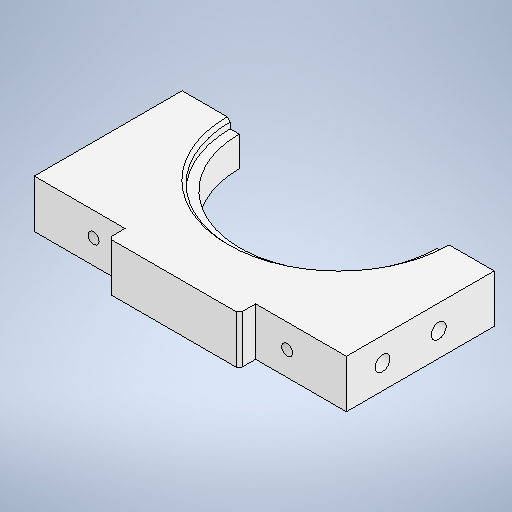
# Autodesk Inventor part: joint4_frame_2
Saved by Autodesk Inventor 2025.3 (Build 293356030, 356C)
## iProperties
Created: 2025-11-09
Part Number: joint4_frame_2
Material: PLA filament
Document SubType Name: Modeling
Designer: MSI
Mass: 66.0962 g
Surface Area: 141.432 cm^2
Volume: 55.0801 cm^3
Density: 1.2 g/cm^3
Appearance: 일반
Author: MSI
Autodesk Inventor part; units mm, degrees
ref_plane "YZ Plane" through (0, 0, 0) normal (1, 0, 0) x (0, 1, 0)
ref_plane "XZ Plane" through (0, 0, 0) normal (0, 1, 0) x (-1, 0, 0)
ref_plane "XY Plane" through (0, 0, 0) normal (0, 0, 1) x (1, 0, 0)
sketch "스케치1" plane through (0, 0, 0) normal (0, 1, 0) x (-1, 0, 0)
  line L0 (-104.5, 55) -> (104.5, 55)
  line L1 (104.5, 55) -> (104.5, -55)
  line L2 (104.5, -55) -> (-104.5, -55)
  line L3 (-104.5, -55) -> (-104.5, 55)
  line L4 (-104.5, 55) -> (104.5, -55) construction
  line L5 (104.5, 55) -> (-104.5, -55) construction
  point P0 (0, 0)
  dimension "d0" = 209
  dimension "d1" = 110
  constraints: 12 end point, 2 midpoint, 2 parallel, 1 horizontal, 1 perpendicular
  measures "d0" distance of L1.end L2.end
  measures "d1" distance of L0.end L1.end
extrude "돌출1" add sketch "스케치1" along normal mid plane 16
sketch "스케치2" plane through (0, 8, 0) normal (0, 1, 0) x (1, 0, 0)
  line L0 (-104.5, 55) -> (-104.5, -55) projected
  line L1 (-104.5, -40) -> (-94, -40)
  line L2 (-94, -40) -> (-94, 40)
  line L3 (-94, 40) -> (-104.5, 40)
  line L4 (-104.5, 40) -> (-104.5, -40)
  line L5 (-104.5, -55) -> (104.5, -55) projected
  point P0 (0, 0)
  point P1 (-94, 0)
  dimension "d4" = 10.5
  dimension "d5" = 15
  constraints: 8 end point, 2 parallel, 1 horizontal, 1 horizontal alignment, 1 midpoint, 1 perpendicular, 1 point on line
  measures "d4" distance of L2.end L3.end
  measures "d5" distance between parallel lines of L5 L1
extrude "돌출2" cut sketch "스케치2" against normal through all
sketch "스케치9" plane through (0, 8, 0) normal (0, 1, 0) x (1, 0, 0)
  line L0 (0, -0.25) -> (-158.4246, -0.25)
  line L1 (-158.4246, -0.25) -> (-158.4246, -70.8007)
  line L2 (-158.4246, -70.8007) -> (0, -70.8007)
  line L3 (0, -70.8007) -> (0, -0.25)
  point P0 (0, 0)
  dimension "d55" = 0.25
  constraints: 8 end point, 2 parallel, 1 horizontal, 1 perpendicular, 1 point on line
  measures "d55" distance from line of point (0, 0) L0
sketch "스케치10" plane through (-35.9991, 8, 0.25) normal (0, 0, -1) x (-1, 0, 0)
  line L0 (6.5004, -8) -> (29.0004, -8)
  line L1 (58.0009, 0) -> (0, 0) projected
  point P0 (-35.9991, -8)
  point P1 (29.0004, 0)
  point P2 (29.0004, 0)
  dimension "d66" = 22.5
  constraints: 2 coincident, 2 end point, 2 midpoint, 1 horizontal, 1 point on line, 1 vertical alignment
  measures "d66" distance of L0.start L0.end
mirror "미러1" about plane through (0, 0, 0) normal (1, 0, 0) of "돌출2"
sketch "스케치3" plane through (-94, 8, -40) normal (-1, 0, 0) x (0, 0, 1)
  line L0 (13.4, -8) -> (66.6, -8)
  point P0 (40, -8)
  point P1 (40, -8)
  point P2 (26.7, -8)
  point P3 (53.3, -8)
  dimension "d8" = 13.3
  dimension "d9" = 13.3
  dimension "d10" = 53.2
  constraints: 3 coincident, 2 end point, 2 point on line, 1 horizontal, 1 midpoint
  measures "d8" distance of point (26.7, -8) point (13.4, -8)
  measures "d9" distance of point (53.3, -8) point (66.6, -8)
  measures "d10" distance of L0.start L0.end
hole "구멍1" at (-94, 0, -26.6) at (-94, 0, -13.3) at (-94, 0, 13.3) at (-94, 0, 26.6) direction (1, 0, 0) diameter 3.6881 depth 13 tip angle 118 thread size "M4.5x0.75" class "6H" standard "ISO Metric profile"
sketch "스케치4" plane through (0, 8, 0) normal (0, 1, 0) x (1, 0, 0)
  line L0 (-99.25, 47.5) -> (-99.25, -47.5)
  line L1 (-94, -40) -> (-104.5, -40) projected
  line L2 (-104.5, -55) -> (104.5, -55) projected
  point P0 (0, 0)
  point P1 (-99.25, 0)
  point P2 (-99.25, -40)
  dimension "d18" = 7.5
  constraints: 2 end point, 2 midpoint, 1 horizontal alignment, 1 point on line, 1 vertical
  measures "d18" distance from line of L0.end L2
hole "구멍2" at (-99.25, 8, 47.5) at (-99.25, 8, -47.5) direction (0, -1, 0) diameter 4.5 end through all counterbore diameter 8 counterbore depth 4.4 clearance for "Socket Head Cap Screw ISO 4762" size "M4" standard "ISO"
mirror "미러2" about plane through (0, 0, 0) normal (1, 0, 0) of "구멍1", "구멍2"
sketch "스케치5" plane through (0, 8, 0) normal (0, 1, 0) x (1, 0, 0)
  point P0 (0, 0)
hole "구멍3" at (0, 8, 0) direction (0, -1, 0) diameter 66 end through all counterbore diameter 72 counterbore depth 3
mirror "미러4" about plane through (0, 0, 0) normal (0, 1, 0) of "구멍3"
sketch "스케치11" plane through (-104.5, 8, 55) normal (0, 0, 1) x (1, 0, 0)
  line L0 (0, 0) -> (209, 0) projected
  line L1 (209, -16) -> (0, -16) projected
  line L2 (21.75, 0) -> (82.75, 0)
  line L3 (82.75, 0) -> (82.75, -16)
  line L4 (82.75, -16) -> (21.75, -16)
  line L5 (21.75, -16) -> (21.75, 0)
  point P0 (104.5, -8)
  point P1 (52.25, 0)
  point P2 (21.75, -16)
  dimension "d68" = 61
  dimension "d69" = 52.25
  constraints: 8 end point, 2 parallel, 2 point on line, 1 horizontal, 1 midpoint, 1 perpendicular
  measures "d68" distance between parallel lines of L3 L5
  measures "d69" horizontal distance of point (104.5, -8) point (52.25, 0)
extrude "돌출5" cut sketch "스케치11" against normal blind 5.5
sketch "스케치6" plane through (-104.5, 8, 49.5) normal (0, 0, 1) x (1, 0, 0)
  line L0 (32.25, -8) -> (72.25, -8)
  point P0 (104.5, -8)
  point P1 (104.5, -8)
  point P2 (52.25, -8)
  dimension "d33" = 40
  dimension "d67" = 52.25
  constraints: 2 end point, 1 coincident, 1 horizontal, 1 midpoint, 1 point on line
  measures "d33" distance of L0.start L0.end
  measures "d67" distance of point (52.25, -8) point (104.5, -8)
hole "구멍4" at (-72.25, 0, 49.5) at (-32.25, 0, 49.5) direction (0, 0, -1) diameter 3.6881 depth 13 tip angle 118 thread size "M4.5x0.75" class "6H" standard "ISO Metric profile"
mirror "미러3" about plane through (0, 0, 0) normal (0, 0, 1) of "구멍4", "돌출5"
mirror "미러5" about plane through (0, 0, 0) normal (1, 0, 0) of "구멍4", "미러3", "돌출5"
chamfer "모따기1" distance 1 angle 45 14 edges at (104.5, 0, -40) (104.5, 0, 40) (21.75, 0, 55) (82.75, 0, 55) (-82.75, 0, 55) (-21.75, 0, 55) (21.75, 0, -55) (82.75, 0, -55) (-82.75, 0, -55) (-21.75, 0, -55) (-104.5, 0, 40) (-104.5, 0, -40) (0, 8, -36) (0, -8, -36)
sketch "스케치7" plane through (0, 0, 0) normal (0, 0, 1) x (1, 0, 0)
  line L0 (-52, -71.98) -> (52, -71.98)
  line L1 (52, -71.98) -> (52, 71.98)
  line L2 (52, 71.98) -> (-52, 71.98)
  line L3 (-52, 71.98) -> (-52, -71.98)
  line L4 (-82.75, 8) -> (-21.75, 8) projected
  line L5 (21.75, 8) -> (82.75, 8) projected
  point P0 (0, 0)
  point P1 (-52, 0)
  point P2 (-52.25, 8)
  point P3 (52.25, 8)
  dimension "d75" = 0.25
  dimension "d76" = 0.25
  constraints: 8 end point, 3 midpoint, 2 parallel, 1 horizontal, 1 horizontal alignment, 1 perpendicular
  measures "d75" distance from line of point (-52.25, 8) L3
  measures "d76" distance from line of point (52.25, 8) L1
extrude "돌출3" cut sketch "스케치7" along normal through all both and the other way through all keep common part
sketch "스케치8" plane through (-52, -8, -55) normal (-1, 0, 0) x (0, 0, -1)
  line L0 (-92.5, -8) -> (-17.5, -8)
  point P0 (-55, -8)
  point P1 (-55, -8)
  point P2 (-73.75, -8)
  point P3 (-36.25, -8)
  dimension "d52" = 18.75
  dimension "d53" = 18.75
  dimension "d54" = 75
  constraints: 3 coincident, 2 end point, 2 point on line, 1 horizontal, 1 midpoint
  measures "d52" distance of point (-73.75, -8) point (-92.5, -8)
  measures "d53" distance of point (-17.5, -8) point (-36.25, -8)
  measures "d54" distance of L0.start L0.end
hole "구멍5" at (-52, 0, 37.5) at (-52, 0, -37.5) at (-52, 0, -18.75) at (-52, 0, 18.75) direction (1, 0, 0) diameter 5 depth 10 tip angle 118
mirror "미러6" about plane through (0, 0, 0) normal (1, 0, 0) of "구멍5"
sketch "스케치12" plane through (0, 0, 0) normal (0, 1, 0) x (-1, 0, 0)
  line L0 (92.3449, 71.8802) -> (-92.3449, 71.8802)
  line L1 (-92.3449, 71.8802) -> (-92.3449, 0.25)
  line L2 (-92.3449, 0.25) -> (92.3449, 0.25)
  line L3 (92.3449, 0.25) -> (92.3449, 71.8802)
  point P0 (0, 0)
  point P1 (0, 0.25)
  dimension "d77" = 0.25
  constraints: 8 end point, 2 parallel, 1 horizontal, 1 midpoint, 1 perpendicular, 1 vertical alignment
  measures "d77" distance from line of point (0, 0) L2
extrude "돌출6" cut sketch "스케치12" along normal through all both and the other way through all keep common part
sketch "스케치13" plane through (-36.9992, -8, 0.25) normal (0, 0, -1) x (-1, 0, 0)
  line L0 (5.5008, 8) -> (-79.4992, 8)
  point P0 (-36.9992, 8)
  point P1 (-36.9992, 8)
  dimension "d80" = 85
  constraints: 3 coincident, 2 end point, 1 horizontal, 1 midpoint
  measures "d80" distance of L0.start L0.end
hole "구멍7" at (-42.5, 0, 0.25) at (42.5, 0, 0.25) direction (0, 0, 1) diameter 5 depth 10 tip angle 118
equation "\"d9\" = d8"
equation "\"d10\" = 4 * d8"
equation "\"d76\" = d75"
equation "\"d53\" = d52"
equation "\"d54\" = 4 * d52"
